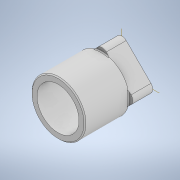
# Autodesk Inventor part: Пункт 1(чё там считать)
Saved by Autodesk Inventor 2021 (Build 250183000, 183)
## iProperties
Created: 2020-05-07
Part Number: Пункт 1(чё там считать)
Material: Типовые
Document SubType Name: Modeling
Designer: 2000
Density: 1 g/cm^3
Appearance: По умолчанию
Mass: 542.726 g
Surface Area: 965.034 cm^2
Volume: 542.726 cm^3
Author: 2000
Autodesk Inventor part; units mm, degrees
ref_plane "YZ Plane" through (0, 0, 0) normal (1, 0, 0) x (0, 1, 0)
ref_plane "XZ Plane" through (0, 0, 0) normal (0, 1, 0) x (-1, 0, 0)
ref_plane "XY Plane" through (0, 0, 0) normal (0, 0, 1) x (1, 0, 0)
sketch "Эскиз1" plane through (0, 0, 0) normal (0, 0, 1) x (1, 0, 0)
  line L0 (-8.4853, 57.9828) -> (-57.9828, 8.4853)
  line L1 (-57.9828, -8.4853) -> (-8.4853, -57.9828)
  line L2 (8.4853, -57.9828) -> (57.9828, -8.4853)
  line L3 (57.9828, 8.4853) -> (8.4853, 57.9828)
  line L4 (-93.0553, 0) -> (93.0553, 0) projected
  line L5 (0, -87.0906) -> (0, 92.0611) projected
  arc A0 (-57.9828, 8.4853) -> (-57.9828, -8.4853) centre (-49.4975, 0) ccw
  arc A1 (8.4853, 57.9828) -> (-8.4853, 57.9828) centre (0, 49.4975) ccw
  arc A2 (57.9828, -8.4853) -> (57.9828, 8.4853) centre (49.4975, 0) ccw
  arc A3 (-8.4853, -57.9828) -> (8.4853, -57.9828) centre (0, -49.4975) ccw
  point P0 (0, 66.468)
  point P1 (-66.468, 0)
  point P2 (66.468, 0)
  dimension "d5" = 94
  dimension "d7" = 94
  dimension "d8" = 12
  constraints: 8 end point, 8 point on circle, 8 point on line, 8 tangent, 4 centre point, 3 equal radius, 2 perpendicular, 1 horizontal alignment, 1 parallel
  measures "d5" distance of point (66.468, 0) point (0, 66.468)
  measures "d7" distance of point (0, 66.468) point (-66.468, 0)
  measures "d8" radius of A0
extrude "Выдавливание1" add sketch "Эскиз1" along normal blind 40
sketch "Эскиз2" plane through (0, 0, 40) normal (0, 0, 1) x (1, 0, 0)
  circle A0 centre (0, 0) radius 54
  dimension "d11" = 108
  constraints: 1 centre point, 1 coincident
  measures "d11" diameter of A0
extrude "Выдавливание2" add sketch "Эскиз2" along normal blind 88
sketch "Эскиз3" plane through (0, 0, 128) normal (0, 0, 1) x (1, 0, 0)
  circle A0 centre (0, 0) radius 42
  dimension "d14" = 84
  constraints: 1 centre point, 1 coincident
  measures "d14" diameter of A0
extrude "Выдавливание3" cut sketch "Эскиз3" against normal blind 79
sketch "Эскиз4" plane through (0, 0, 0) normal (0, 0, -1) x (-1, 0, 0)
  circle A0 centre (0, 0) radius 36
  dimension "d17" = 72
  constraints: 1 centre point, 1 coincident
  measures "d17" diameter of A0
extrude "Выдавливание4" cut sketch "Эскиз4" against normal blind 40
chamfer "Фаска1" distance 2 angle 45 1 edges at (-54, 0, 128)
chamfer "Фаска2" distance 1.6 angle 45 1 edges at (36, 0, 0)
sketch "Эскиз6" plane through (0, 0, 0) normal (0, 0, -1) x (-1, 0, 0)
  circle A0 centre (0, 49) radius 6
  circle A1 centre (0, -49) radius 6
  line L0 (86.0965, 0) -> (-86.0965, 0) projected
  circle A2 centre (49, 0) radius 6
  circle A3 centre (-49, 0) radius 6
  line L1 (0, -86.0965) -> (0, 86.0965) projected
  point P0 (0, 0)
  dimension "d30" = 98
  dimension "d31" = 12
  dimension "d32" = 12
  dimension "d33" = 98
  dimension "d34" = 12
  dimension "d35" = 12
  constraints: 4 centre point, 2 point on line, 2 symmetric about line
  measures "d30" distance of A1.centre A0.centre
  measures "d31" diameter of A1
  measures "d32" diameter of A0
  measures "d33" distance of A2.centre A3.centre
  measures "d34" diameter of A2
  measures "d35" diameter of A3
fillet "Сопряжение1" radius 2 5 edges at (0, 54, 40) (-54, 0, 40) (0, -54, 40) (53.5066, -7.2827, 40) (53.5066, 7.2827, 40)
hole "Отверстие1" at (49, 0, 0) direction (0, 0, 1) diameter 10.106 depth 30.5 tip angle 118 thread size "M12x1.75" class "6H" standard "ANSI Metric M Profile"
chamfer "Фаска3" distance 2 angle 45 1 edges at (49, -5.053, 0)
sketch "Эскиз7" plane through (0, 0, 0) normal (0, 0, -1) x (-1, 0, 0)
  circle A0 centre (49, 0) radius 6
  point P0 (0, 0)
  dimension "d47" = 49
  dimension "d48" = 12
  constraints: 1 centre point
  measures "d47" distance of A0.centre point (0, 0)
  measures "d48" diameter of A0
hole "Отверстие2" at (-49, 0, 0) direction (0, 0, 1) diameter 10.106 depth 30.5 tip angle 118 thread size "M12x1.75" class "6H" standard "ANSI Metric M Profile"
chamfer "Фаска4" distance 2 angle 45 1 edges at (-49, -5.053, 0)
sketch "Эскиз8" plane through (0, 0, 0) normal (0, 0, -1) x (-1, 0, 0)
  circle A0 centre (0, 49) radius 6
  point P0 (0, 0)
  dimension "d59" = 12
  dimension "d60" = 49
  constraints: 1 centre point
  measures "d59" diameter of A0
  measures "d60" distance of point (0, 0) A0.centre
hole "Отверстие3" at (0, 49, 0) direction (0, 0, 1) diameter 10.106 depth 30.5 tip angle 118 thread size "M12x1.75" class "6H" standard "ANSI Metric M Profile"
chamfer "Фаска5" distance 2 angle 45 1 edges at (0, 43.947, 0)
sketch "Эскиз9" plane through (0, 0, 0) normal (0, 0, -1) x (-1, 0, 0)
  circle A0 centre (0, -49) radius 6
  point P0 (0, 0)
  dimension "d71" = 12
  dimension "d72" = 49
  constraints: 1 centre point
  measures "d71" diameter of A0
  measures "d72" distance of point (0, 0) A0.centre
hole "Отверстие4" at (0, -49, 0) direction (0, 0, 1) diameter 10.106 depth 30.5 tip angle 118 thread size "M12x1.75" class "6H" standard "ANSI Metric M Profile"
chamfer "Фаска6" distance 2 angle 45 1 edges at (0, -54.053, 0)
